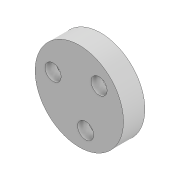
# Autodesk Inventor part: Cover of gearbox 2
Saved by Autodesk Inventor 2020.3 (Build 243373010, 373A)
## iProperties
Created: 2021-05-03
Part Number: Cover of gearbox 2
Material: Generic
Document SubType Name: Modeling
Designer: marti
Density: 1 g/cm^3
Appearance: Default
Author: marti
Autodesk Inventor part; units mm, degrees
ref_plane "YZ Plane" through (0, 0, 0) normal (1, 0, 0) x (0, 1, 0)
ref_plane "XZ Plane" through (0, 0, 0) normal (0, 1, 0) x (-1, 0, 0)
ref_plane "XY Plane" through (0, 0, 0) normal (0, 0, 1) x (1, 0, 0)
sketch "Sketch1" plane through (0, 0, 0) normal (0, 0, 1) x (1, 0, 0)
  circle A0 centre (-24.4499, 7.2424) radius 7.5
  circle A1 centre (18.497, 17.553) radius 7.5
  circle A2 centre (5.9529, -24.7954) radius 7.5
  circle A3 centre (0, 0) radius 40
  circle A4 centre (0, 0) radius 41.25
  point P0 (0, 0)
  dimension "d9" = 82.5
  constraints: 5 centre point, 1 coincident
  measures "d9" diameter of A4
extrude "Extrusion1" add sketch "Sketch1" against normal blind 20 contours A3 | A4
sketch "Sketch4" plane through (0, 0, -20) normal (0, 0, -1) x (-1, 0, 0)
  circle A0 centre (0, 0) radius 41.25 projected
  circle A1 centre (0, 0) radius 40
  point P0 (0, 0)
  dimension "d10" = 80
  constraints: 1 centre point, 1 coincident
  measures "d10" diameter of A1
extrude "Extrusion4" cut sketch "Sketch4" against normal blind 10 contours A1
body "Solid1"
